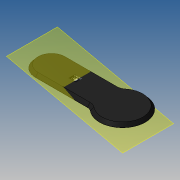
# Autodesk Inventor part: gornji shiny dio
Saved by Autodesk Inventor 2014 (Build 180170000, 170)
## iProperties
Created: 2011-11-30
Part Number: gornji shiny dio
Material: Generic
Document SubType Name: Modeling
Designer: slazh bliskovic
Density: 1 g/cm^3
Mass: 4.94251 g
Surface Area: 46.167 cm^2
Volume: 4.94251 cm^3
Appearance: Glossy - Black
Author: slazh bliskovic
Autodesk Inventor part; units mm, degrees
ref_plane "YZ Plane" through (0, 0, 0) normal (1, 0, 0) x (0, 1, 0)
ref_plane "XZ Plane" through (0, 0, 0) normal (0, 1, 0) x (-1, 0, 0)
ref_plane "XY Plane" through (0, 0, 0) normal (0, 0, 1) x (1, 0, 0)
sketch "Sketch1" plane through (0, 0, 0) normal (0, 0, 1) x (1, 0, 0)
  spline S0 degree 3 poles (12.7758, 13.7437) (13.4536, 14.296) (14.1651, 14.793) (16.9373, 16.4418) (19.2243, 17.2436) (24.5957, 17.9791) (27.7237, 17.5963) (32.8694, 15.5351) (34.9647, 14.1297) (38.6283, 10.3594) (40.0896, 7.8966) (41.4354, 3.545) (41.7033, 1.7728) (41.7033, 0) (41.7033, -1.7729) (41.4354, -3.5451) (40.0895, -7.897) (38.6278, -10.3602) (34.9655, -14.1286) (32.8727, -15.5328) (27.7225, -17.598) (24.5861, -17.9808) (19.2198, -17.2406) (16.945, -16.4433) (14.1759, -14.8006) (13.4587, -14.3002) (12.7758, -13.7437) knots 0.047577 0.047577 0.047577 0.047577 0.308418 0.308418 1.015437 1.015437 1.927825 1.927825 2.666741 2.666741 3.497446 3.497446 4.02653 4.02653 4.02653 4.555615 4.555615 5.386442 5.386442 6.124601 6.124601 7.039356 7.039356 7.74266 7.74266 8.00548 8.00548 8.00548 8.00548 weights 1 1 1 1 1 1 1 1 1 1 1 1 1 1 1 1 1 1 1 1 1 1 1 1 1 1 1
  spline S1 degree 3 poles (12.7758, -13.7437) (12.3265, -13.3776) (11.8219, -13.0794) (10.6568, -12.62) (9.9847, -12.4901) (9.3118, -12.4901) knots 0 0 0 0 0.462707 0.462707 1 1 1 1 weights 1 1 1 1 1 1
  line L0 (9.3118, -12.4901) -> (-31.0253, -12.4901)
  spline S2 degree 3 poles (9.3118, 12.4901) (9.7991, 12.4901) (10.2862, 12.5578) (11.492, 12.896) (12.1826, 13.2604) (12.7758, 13.7437) knots 0 0 0 0 0.389114 0.389114 1 1 1 1 weights 1 1 1 1 1 1
  line L1 (0, 0) -> (-42.2873, 0) construction
  line L2 (9.3118, 12.4901) -> (-31.0253, 12.4901)
  arc A0 (-31.0253, 12.4901) -> (-31.0253, -12.4901) centre (-31.0253, 0) ccw
  constraints: 2 end point, 2 point on circle, 1 centre point, 1 parallel, 1 point on line, 1 symmetric about line
extrude "Extrusion1" add sketch "Sketch1" along normal blind 2.5
chamfer "Chamfer1" distance 2 angle 50 6 edges at (41.7033, 0, 2.5) (11.1518, -12.8172, 2.5) (-10.8568, -12.4901, 2.5) (-43.5155, 0, 2.5) (-10.8568, 12.4901, 2.5) (11.1517, 12.8172, 2.5) measured on face at (-4.1339, -4.1634, 2.5)
sketch "Sketch6" plane through (0, 0, 2.5) normal (0, 0, 1) x (1, 0, 0)
  line L0 (-9.5253, -2.5425) -> (-15.3564, -2.5425) construction
  line L1 (-15.3564, -2.5425) -> (-15.3564, 2.5425) construction
  line L2 (-15.3564, 2.5425) -> (-9.5253, 2.5425) construction
  line L3 (-9.5253, 2.5425) -> (-9.5253, -2.5425) construction
  point P0 (0, 0)
  point P1 (-6.2263, 0)
  constraints: 1 horizontal alignment, 2 other
decal "Decal1"
ref_plane "Work Plane1" through (0, 0, 0) normal (0.2164396, 0, 0.976296) x (0, 1, 0)
sketch "Sketch7" plane through (0, 0, 0) normal (0.2164396, 0, 0.976296) x (0, 1, 0)
  point P0 (0, 0)
ref_plane "Work Plane2" through (0, 0, 0) normal (0.2164396, 0, 0.976296) x (0, 1, 0)
body "Solid1"
